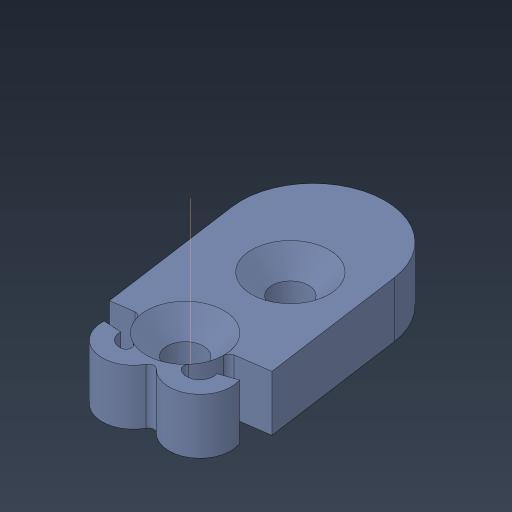
# Autodesk Inventor part: Dribbler Slider
Saved by Autodesk Inventor 2023.1 (Build 271208000, 208)
## iProperties
Part Number: Dribbler Slider
Material: Gummi, Silikon
Document SubType Name: Modeling
Designer: rYan
Mass: 1.05946 g
Surface Area: 7.33408 cm^2
Volume: 0.847566 cm^3
Density: 1.25 g/cm^3
Appearance: Gummi - Blau
Author: rYan
Autodesk Inventor part; units mm, degrees
ref_plane "YZ Plane" through (0, 0, 0) normal (1, 0, 0) x (0, 1, 0)
ref_plane "XZ Plane" through (0, 0, 0) normal (0, 1, 0) x (-1, 0, 0)
ref_plane "XY Plane" through (0, 0, 0) normal (0, 0, 1) x (1, 0, 0)
sketch "Skizze1" plane through (0, 0, 0) normal (0, 0, 1) x (1, 0, 0)
  line L0 (0.5, 0) -> (-1.3093, 12.8735) construction
  line L1 (6.9367, 0.9046) -> (5.1275, 13.7781)
  line L2 (-7.746, 11.9689) -> (-5.9367, -0.9046)
  arc A0 (-5.9367, -0.9046) -> (6.9367, 0.9046) centre (0.5, 0) ccw
  arc A1 (5.1275, 13.7781) -> (-7.746, 11.9689) centre (-1.3093, 12.8735) ccw
  line L3 (0, 0) -> (0, 9.5) construction
  line L4 (5, -11) -> (-5, -11) construction
  line L5 (0, 0) -> (0, -11) construction
  line L6 (-8.5, 9.1711) -> (-8.5, -11) construction
  dimension "d0" = 13
  dimension "d1" = 13
  dimension "d14" = 9.5
  dimension "d17" = 8
  dimension "d26" = 11
  dimension "d27" = 10
  dimension "d28" = 11
  dimension "d29" = 8.5
  dimension "d30" = 9
  constraints: 16 end point, 4 point on circle, 4 tangent, 3 coincident, 3 vertical, 2 centre point, 1 horizontal, 1 midpoint, 1 parallel, 1 point on line
  measures "d0" diameter of A1
  measures "d1" distance of L0.start L0.end
  measures "d14" distance of L3.start L3.end
  measures "d17" angle of L0 L3
  measures "d26" distance from line of L4 L3.start
  measures "d27" distance of L4.start L4.end
  measures "d28" distance from line of L4 L0.start
  measures "d29" distance between parallel lines of L6 L3
  measures "d30" distance from line of L0.start L6
extrude "Extrusion1" add sketch "Skizze1" against normal blind 5
hole "Bohrung2" at (0, 9.5, 0) at (0, 0, 0) direction (0, 0, -1) diameter 3.3 end through all countersink diameter 7 countersink angle 90
sketch "Skizze4" plane through (0, 0, 0) normal (0, 0, 1) x (1, 0, 0)
  circle A0 centre (0, 0) radius 3.5 projected
  arc A1 (2.3743, -2.5715) -> (4.6334, -1.7614) centre (3.5024, -2.1623) ccw
  arc A2 (0.9725, -3.3622) -> (6.1415, -1.2268) centre (3.5024, -2.1623) ccw
  arc A3 (-5.9367, -0.9046) -> (6.9367, 0.9046) centre (0.5, 0) ccw projected
  line L0 (4.6334, -1.7614) -> (6.1415, -1.2268)
  line L1 (-5.9367, -0.9046) -> (6.9367, 0.9046)
  line L2 (0.5, 0) -> (1.4046, -6.4367) construction
  arc A4 (-4.5848, -2.7343) -> (0.9725, -3.3622) centre (-1.7901, -2.9061) ccw
  arc A5 (-2.9878, -2.8325) -> (-0.7092, -3.4274) centre (-1.7901, -2.9061) ccw
  line L3 (-2.9878, -2.8325) -> (-4.5848, -2.7343)
  point P0 (-3.4556, -0.5559)
  point P1 (-3.5231, -5.1053)
  point P2 (5.7745, -3.7986)
  point P3 (3.4749, 0.4181)
  dimension "d38" = 1.2
  dimension "d39" = 1.6
  dimension "d40" = 2
  dimension "d41" = 1.6
  dimension "d42" = 1.2
  dimension "d43" = 2
  constraints: 12 point on circle, 8 end point, 4 centre point, 3 point on line, 2 coincident, 2 tangent, 1 perpendicular
  measures "d38" radius of A1
  measures "d39" radial gap between concentric circles of A1 A2
  measures "d40" distance from line of L1 L0.end
  measures "d41" radial gap between concentric circles of A5 A4
  measures "d42" radius of A5
  measures "d43" distance from line of L3.end L1
extrude "Extrusion3" cut sketch "Skizze4" against normal through all contours A5 L3 A4 A3 L1 A0 | A2 A3 A4 | A0 L1 A3 A2 L0 A1
fillet "Rundung2" radius 0.5 5 edges at (-3.4556, -0.5559, -2.5) (3.4749, 0.4181, -2.5) (2.3743, -2.5715, -2.5) (-0.7092, -3.4274, -2.5) (0.9725, -3.3622, -2.5)
equation "\"d28\" = d_Boden"
equation "\"d30\" = d_Vorne"
equation "\"d41\" = d39"
equation "\"d42\" = d38"
equation "\"d43\" = d40"
equation "\"d_Boden\" = 11"
equation "\"d_Vorne\" = 9"
